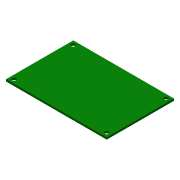
# Autodesk Inventor part: MainBoard
Saved by Autodesk Inventor 2015 (Build 190159000, 159)
## iProperties
Created: 2013-01-19
Part Number: MainBoard
Material: Silicon Nitride
Document SubType Name: Modeling
Designer: davidgitz
Density: 1 g/cm^3
Appearance: Dark Green
Author: davidgitz
Autodesk Inventor part; units mm, degrees
ref_plane "YZ Plane" through (0, 0, 0) normal (1, 0, 0) x (0, 1, 0)
ref_plane "XZ Plane" through (0, 0, 0) normal (0, 1, 0) x (-1, 0, 0)
ref_plane "XY Plane" through (0, 0, 0) normal (0, 0, 1) x (1, 0, 0)
sketch "Sketch1" plane through (0, 0, 0) normal (0, 1, 0) x (-1, 0, 0)
  line L0 (-38.227, 25.527) -> (38.227, 25.527)
  line L1 (38.227, 25.527) -> (38.227, -25.527)
  line L2 (38.227, -25.527) -> (-38.227, -25.527)
  line L3 (-38.227, -25.527) -> (-38.227, 25.527)
  line L4 (-38.227, 25.527) -> (38.227, -25.527) construction
  point P0 (0, 0)
  point P1 (0, 0)
  dimension "d0" = 76.454
  dimension "d1" = 51.054
  constraints: 10 end point, 2 parallel, 1 coincident, 1 horizontal, 1 midpoint, 1 perpendicular
  measures "d0" distance of L1.end L2.end
  measures "d1" distance of L0.end L1.end
extrude "Extrusion1" add sketch "Sketch1" along normal blind 1.524
sketch "Sketch2" plane through (0, 1.524, 0) normal (0, 1, 0) x (1, 0, 0)
  line L0 (-38.227, -25.527) -> (38.227, -25.527) projected
  line L1 (38.227, -25.527) -> (38.227, 25.527) projected
  line L2 (38.227, 25.527) -> (-38.227, 25.527) projected
  line L3 (-38.227, 25.527) -> (-38.227, -25.527) projected
  circle A0 centre (-35.179, 22.479) radius 1.524
  circle A1 centre (-35.179, -22.479) radius 1.524
  circle A2 centre (35.179, 22.479) radius 1.524
  circle A3 centre (35.179, -22.479) radius 1.524
  point P0 (0, 0)
  dimension "d4" = 3.048
  dimension "d5" = 3.048
  dimension "d6" = 3.048
  dimension "d7" = 3.048
  dimension "d8" = 3.048
  dimension "d9" = 3.048
  dimension "d10" = 3.048
  dimension "d11" = 3.048
  dimension "d12" = 3.048
  constraints: 4 centre point, 3 equal radius
  measures "d4" diameter of A0
  measures "d5" distance from line of A0.centre L2
  measures "d6" distance from line of L3 A0.centre
  measures "d7" distance from line of L3 A1.centre
  measures "d8" distance from line of L0 A1.centre
  measures "d9" distance from line of L2 A2.centre
  measures "d10" distance from line of A2.centre L1
  measures "d11" distance from line of L1 A3.centre
  measures "d12" distance from line of L0 A3.centre
extrude "Extrusion2" cut sketch "Sketch2" against normal up to next contours A0 | A1 | A2 | A3
body "Solid1"
